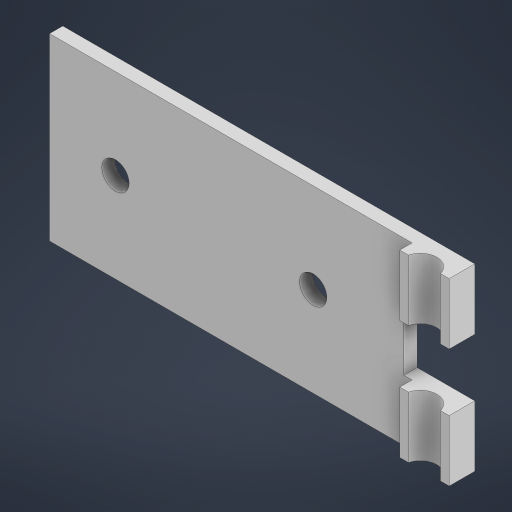
# Autodesk Inventor part: Counter
Saved by Autodesk Inventor 2024.2 (Build 282272000, 272)
## iProperties
Created: 2024-06-05
Part Number: Counter
Material: Generic
Document SubType Name: Modeling
Designer: simon
Density: 1 g/cm^3
Appearance: Default
Author: simon
Autodesk Inventor part; units mm, degrees
ref_plane "YZ Plane" through (0, 0, 0) normal (1, 0, 0) x (0, 1, 0)
ref_plane "XZ Plane" through (0, 0, 0) normal (0, 1, 0) x (-1, 0, 0)
ref_plane "XY Plane" through (0, 0, 0) normal (0, 0, 1) x (1, 0, 0)
sketch "Sketch1" plane through (0, 0, 0) normal (0, 0, 1) x (1, 0, 0)
  line L0 (0, 0) -> (50, 0)
  line L1 (50, 0) -> (50, 21.8)
  line L2 (50, 21.8) -> (0, 21.8)
  line L3 (0, 21.8) -> (0, 0)
  circle A0 centre (8, 10.9) radius 1.65
  circle A1 centre (32, 10.9) radius 1.65
  line L4 (50, 14.4) -> (43, 14.4)
  line L5 (43, 14.4) -> (43, 7.4)
  line L6 (43, 7.4) -> (50, 7.4)
  line L7 (50, 7.4) -> (50, 14.4)
  point P0 (46.5, 14.4)
  dimension "d0" = 50
  dimension "d1" = 21.8
  dimension "d2" = 3.3
  dimension "d3" = 3.3
  dimension "d4" = 8
  dimension "d5" = 24
  dimension "d6" = 10.9
  dimension "d7" = 10.9
  dimension "d10" = 7
  dimension "d11" = 7
  dimension "d12" = 7.4
  constraints: 16 end point, 4 parallel, 2 centre point, 2 horizontal, 2 perpendicular, 1 midpoint, 1 point on line
  measures "d0" distance of L2.end L1.end
  measures "d1" distance of L1.end L0.end
  measures "d2" diameter of A0
  measures "d3" diameter of A1
  measures "d4" distance from line of A0.centre L3
  measures "d5" distance of A1.centre A0.centre
  measures "d6" distance from line of L2 A0.centre
  measures "d7" distance from line of L2 A1.centre
  measures "d10" distance of L6.end L5.end
  measures "d11" distance of L5.end L4.end
  measures "d12" distance from line of L2 point (46.5, 14.4)
extrude "Extrusion1" add sketch "Sketch1" along normal blind 1.6 contours L3 L2 L1 L4 L5 L6 L0
sketch "Sketch2" plane through (0, 0, 0) normal (0, -1, 0) x (1, 0, 0)
  line L0 (50, 0) -> (50, 1.6) projected
  line L1 (50, 1.6) -> (44, 1.6)
  line L2 (44, 1.6) -> (44, 3.1)
  line L3 (44, 3.1) -> (50, 3.1)
  line L4 (50, 3.1) -> (50, 1.6)
  circle A0 centre (47, 3.6) radius 2
  point P0 (0, 0)
  point P1 (47, 1.6)
  point P2 (47, 1.6)
  point P3 (45.0635, 3.1)
  point P4 (48.9365, 3.1)
  dimension "d13" = 6
  dimension "d14" = 1.5
  dimension "d15" = 4
  dimension "d16" = 2
  dimension "d17" = 3
  constraints: 8 end point, 2 parallel, 1 centre point, 1 horizontal, 1 midpoint, 1 perpendicular
  measures "d13" distance of L2.end L3.end
  measures "d14" distance of L1.end L2.end
  measures "d15" diameter of A0
  measures "d16" distance of point (47, 1.6) A0.centre
  measures "d17" distance from line of A0.centre L4
extrude "Extrusion2" add sketch "Sketch2" against normal blind 21.8 contours L1 A0 L3 L4 | L1 L2 L3 A0
sketch "Sketch3" plane through (0, 0, 1.6) normal (0, 0, 1) x (1, 0, 0)
  line L0 (50, 7.4) -> (50, 14.4) projected
  line L1 (43, 14.4) -> (50, 14.4)
  line L2 (50, 14.4) -> (50, 7.4)
  line L3 (50, 7.4) -> (43, 7.4)
  line L4 (43, 7.4) -> (43, 14.4)
  point P0 (0, 0)
  constraints: 8 end point, 2 parallel, 1 horizontal, 1 perpendicular
extrude "Extrusion3" cut sketch "Sketch3" along normal blind 5 and the other way blind 5
body "Solid1"
